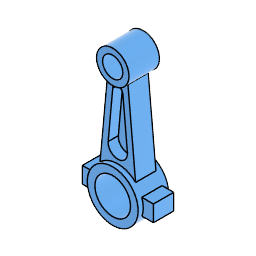
model (Autodesk Fusion 360 design; units mm, degrees)
part number: 2025-08-23-14-37-39-994
Autodesk Fusion 360 part; units mm, degrees
sketch "Sketch1" plane through (0, 0, 0) normal (0, 1, 0) x (1, 0, 0)
  circle A0 centre (0, 0) radius 17.5
  circle A1 centre (0, 0) radius 25
  circle A2 centre (0, -110) radius 10
  circle A3 centre (0, -110) radius 16
  line L0 (-10, -97.51) -> (-17.5, -17.8536)
  line L1 (10, -97.51) -> (17.5, -17.8536)
  line L2 (-23.0003, 9.7972) -> (-34.9353, 9.7972)
  line L3 (-34.9353, 9.7972) -> (-34.9353, -6.2028)
  line L4 (-14.9353, 9.7972) -> (-34.9353, -6.2028) construction
  line L5 (-34.9353, 9.7972) -> (-14.9353, -6.2028) construction
  line L6 (34.9986, -8.2633) -> (34.9986, 7.7367)
  line L7 (34.9986, 7.7367) -> (14.9986, -8.2633) construction
  line L8 (14.9986, 7.7367) -> (34.9986, -8.2633) construction
  line L9 (-34.9353, -6.2028) -> (-24.2183, -6.2028)
  line L10 (23.5949, -8.2633) -> (34.9986, -8.2633)
  line L11 (34.9986, 7.7367) -> (23.7727, 7.7367)
  arc A4 (9.4582, -39.2577) -> (-9.4582, -39.2577) centre (0, -38.3672) ccw
  arc A5 (-4.978, -86.8411) -> (4.978, -86.8411) centre (0, -86.3724) ccw
  line L12 (-4.978, -86.8411) -> (-9.4582, -39.2577)
  line L13 (4.978, -86.8411) -> (9.4582, -39.2577)
  point P0 (-24.9353, 1.7972)
  point P1 (24.9986, -0.2633)
  dimension "d1" = 35
  dimension "d2" = 50
  dimension "d3" = 20
  dimension "d4" = 32
  dimension "d5" = 110
  dimension "d6" = 20
  dimension "d7" = 35
  dimension "d10" = 5
  dimension "d11" = 9.5
  dimension "d12" = 16
  dimension "d13" = 20
  dimension "d14" = 16
  dimension "d15" = 20
  constraint coincident A0.centre A1.centre
  constraint concentric A2 A3
  constraint coincident A3 L0.start
  constraint coincident A1 L0.end
  constraint coincident A3 L1.start
  constraint coincident A1 L1.end
  constraint horizontal L0.start L1.start
  constraint horizontal L0.end L1.end
  constraint horizontal L2
  constraint perpendicular L2 L3
  constraint parallel L2 L9
  constraint coincident L4 P0
  constraint coincident L5 P0
  constraint coincident A1 P0
  constraint horizontal L11
  constraint coincident L7 P1
  constraint coincident L8 P1
  constraint coincident A1 P1
  constraint coincident A1 L9.end
  constraint coincident A1 L2.start
  constraint coincident A1 L10.start
  constraint coincident A1 L11.end
  measures "d1" diameter of A0
  measures "d2" diameter of A1
  measures "d3" diameter of A2
  measures "d4" diameter of A3
  measures "d5" distance of A0.centre A2.centre
  measures "d6" distance of L0.start L1.start
  measures "d7" distance of L0.end L1.end
  measures "d10" radius of A5
  measures "d11" radius of A4
  measures "d12" distance of L2 L9
  measures "d13" distance of L3.end L5.end
  measures "d14" distance of L6.end L6.start
  measures "d15" distance of L6.end L8.start
extrude "Extrude1" add sketch "Sketch1" along normal mid plane 30 contours A1 | A3 makes body 1 at (17.413, 10, 1.7424) makes body 2 at (15.9205, 5, 108.4069)
extrude "Extrude2" add sketch "Sketch1" along normal mid plane 20 contours A1 L6 L10 L11 | A1 L2 L3 L9 | A1 A3 L0 L1 bodies 1 2
extrude "Extrude3" add sketch "Sketch1" along normal blind 8 contours A4 A5 L12 L13 bodies 1
